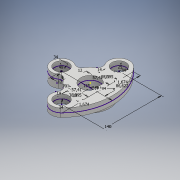
# Autodesk Inventor part: zad6.5-1
Saved by Autodesk Inventor 2018 (Build 220112000, 112)
## iProperties
Created: 2020-04-06
Part Number: zad6.5-1
Material: Типовые
Document SubType Name: Modeling
Designer: Аня
Density: 1 g/cm^3
Appearance: По умолчанию
Author: Аня
Autodesk Inventor part; units mm, degrees
ref_plane "YZ Plane" through (0, 0, 0) normal (1, 0, 0) x (0, 1, 0)
ref_plane "XZ Plane" through (0, 0, 0) normal (0, 1, 0) x (-1, 0, 0)
ref_plane "XY Plane" through (0, 0, 0) normal (0, 0, 1) x (1, 0, 0)
sketch "Эскиз1" plane through (0, 0, 0) normal (0, 0, 1) x (1, 0, 0)
  arc A0 (17, 15.4919) -> (17, -15.4919) centre (0, 0) ccw
  arc A1 (-40.4104, -24) -> (-40.4104, 24) centre (0, 0) ccw
  circle A2 centre (0, -70) radius 17
  circle A3 centre (0, 70) radius 17
  line L0 (0, 0) -> (-70, 0)
  arc A4 (-57.0704, 20.2194) -> (-57.0704, -20.2194) centre (-70, 0) ccw
  circle A5 centre (-70, 0) radius 17
  arc A6 (-57.0704, 20.2194) -> (-40.4104, 24) centre (-50.6056, 30.3291) ccw
  arc A7 (-40.4104, -24) -> (-57.0704, -20.2194) centre (-50.6056, -30.3291) ccw
  arc A8 (-22, -58.1257) -> (-25, -39.7995) centre (-33.8403, -50.6553) ccw
  arc A9 (-25, 39.7995) -> (-22, 58.1257) centre (-33.8403, 50.6553) ccw
  line L1 (0, 0) -> (17, 0)
  line L2 (17, 0) -> (17, -15.4919)
  line L3 (17, 0) -> (17, 15.4919)
  arc A10 (17, -88.3303) -> (17, 88.3303) centre (-71.4464, 0) ccw
  arc A11 (-21.3952, -57.0676) -> (18.6741, -86.6216) centre (0, -70) ccw
  arc A12 (18.6741, 86.6216) -> (-21.3952, 57.0676) centre (0, 70) ccw
  dimension "d0" = 46
  dimension "d1" = 94
  dimension "d2" = 70
  dimension "d5" = 34
  dimension "d6" = 34
  dimension "d10" = 48
  dimension "d11" = 34
  dimension "d12" = 12
  dimension "d13" = 12
  dimension "d14" = 14
  dimension "d15" = 14
  dimension "d17" = 17
  dimension "d18" = 125
  dimension "d19" = 140
  dimension "d20" = 25
  dimension "d21" = 1.6741
  dimension "d22" = 86.6216
  dimension "d23" = 1.6741
  dimension "d24" = 38.3952
  dimension "d25" = 38.3952
  dimension "d26" = 39
  dimension "d27" = 39
  dimension "d28" = 57.4104
  dimension "d29" = 57.4104
  constraints: 30 point on circle, 13 centre point, 8 end point, 6 coincident, 4 tangent, 2 horizontal, 1 equal radius, 1 perpendicular, 1 vertical
  measures "d0" diameter of A0
  measures "d1" diameter of A1
  measures "d2" distance of L0.start L0.end
  measures "d5" diameter of A2
  measures "d6" diameter of A3
  measures "d10" diameter of A4
  measures "d11" diameter of A5
  measures "d12" radius of A6
  measures "d13" radius of A7
  measures "d14" radius of A8
  measures "d15" radius of A9
  measures "d17" distance of L0.start L1.end
  measures "d18" radius of A10
  measures "d19" distance of A2.centre A3.centre
  measures "d20" radius of A12
  measures "d21" distance from line of A12.start L3
  measures "d22" distance from line of A12.start L1
  measures "d23" distance from line of A11.end L3
  measures "d24" distance from line of A12.end L3
  measures "d25" distance from line of A11.start L3
  measures "d26" distance from line of A9.end L3
  measures "d27" distance from line of A8.start L3
  measures "d28" distance from line of A1.end L3
  measures "d29" distance from line of A1.start L3
extrude "Выдавливание1" add sketch "Эскиз1" along normal blind 10 contours A7 A4 A6 A1 | A1 A9 A12 A10 A11 A8
sketch "Эскиз2" plane through (0, 0, 10) normal (0, 0, 1) x (1, 0, 0)
  point P0 (0, 0)
extrude "Выдавливание4" add sketch "Эскиз1" against normal blind 10 contours A1 A9 A12 A10 A11 A8
extrude "Выдавливание5" add sketch "Эскиз1" against normal blind 20 contours A7 A4 A6 A1
